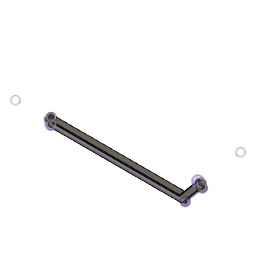
pret_collective (Autodesk Fusion 360 design; units mm, degrees)
part number: 2026-02-12-13-27-31-930
Autodesk Fusion 360 part; units mm, degrees
note: some values were not read from the file. Set by a fixed rule: which sketch regions a step uses.
sketch "Szkic1" plane through (0, 0, 0) normal (0, 1, 0) x (1, 0, 0)
  line L0 (53.834231, -5) -> (-56.165769, -5)
  line L1 (-56.165769, -5) -> (-56.165769, 0)
  line L2 (-56.165769, 0) -> (56.165769, 0)
  line L3 (0, -1.75) -> (0, -22.5)
  line L4 (1.75, 0) -> (22.5, 0)
  line L5 (53.834231, -5) -> (66.689983, -20.320889)
  line L6 (66.689983, -20.320889) -> (70.520205, -17.106951)
  line L7 (70.520205, -17.106951) -> (56.165769, 0)
  dimension "d2" = 110
  dimension "d5" = 5
  dimension "d6" = 130
  dimension "d7" = 20
  dimension "d8" = 5
  constraint perpendicular L0 L1
  constraint collinear L2 L4
  constraint perpendicular L5 L6
  constraint perpendicular L6 L7
  constraint perpendicular L1 L2
  measures "d5" distance of L5 L7
  measures "d6" angle of L0 L5
  measures "d8" distance of L0 L2
extrude "Wyciągnięcie proste1" add sketch "Szkic1" along normal mid plane 6
sketch "Szkic2" plane through (0, 0, 0) normal (0, 1, 0) x (1, 0, 0)
  circle A0 centre (69.890669, -20.246009) radius 1.7
  line L0 (70.520205, -17.106951) -> (66.689983, -20.320889)
  line L1 (68.605094, -18.71392) -> (102.400608, -58.989845)
  line L2 (56.165769, 0) -> (70.520205, -17.106951)
  line L3 (68.227373, -20.597355) -> (67.456027, -19.678101)
  line L4 (70.525506, -18.668992) -> (69.754161, -17.749738)
  line L5 (-57.365769, -4) -> (-56.165769, -4)
  circle A1 centre (-58.165769, -2.5) radius 1.7
  line L6 (-56.165769, -5) -> (-56.165769, 0)
  line L7 (-56.165769, -2.5) -> (-86.029119, -2.5)
  line L8 (-57.365769, -1) -> (-56.165769, -1)
  line L9 (-56.165769, 0) -> (56.165769, 0)
  point P0 (-56.165769, -5)
  dimension "d9" = 3.4
  dimension "d12" = 3
  dimension "d13" = 2
  dimension "d14" = 3.4
  dimension "d15" = 3
  dimension "d16" = 2
  constraint parallel L1 L2
  constraint perpendicular L0 L3
  constraint perpendicular L0 L4
  constraint symmetric L1 L3 L4
  constraint perpendicular L6 L8
  constraint perpendicular L5 L6
  constraint symmetric L5 L7 L8
  constraint vertical L6
  measures "d9" diameter of A0
  measures "d12" distance of L3 L4
  measures "d14" diameter of A1
  measures "d15" distance of L5 L8
revolve "Obrót1" add sketch "Szkic2" angle 360 about axis through (-56.165769, 0, 2.5) along (-1, 0, 0) contours L5 A1 L6 L7 | A1 L7 picked at (-56.286331, -3.151262) picked at (-58.215553, -3.147012)
revolve "Obrót2" add sketch "Szkic2" angle 360 about axis through (68.605094, 0, 18.71392) along (0.642788, 0, 0.766044) contours A0 L1 | A0 L0 L1 L3 picked at (69.144793, -20.686225) picked at (68.183694, -19.224899)
fillet "Zaokrąglenie1" radius 0.5 16 edges at (-1.165769, 3, 5) (0, 3, 0) (60.262107, -3, 12.660444) (60.262107, 3, 12.660444) (63.342987, -3, 8.553475) (63.342987, 3, 8.553475) (-1.165769, -3, 5) (0, -3, 0) (70.520205, 0, 17.106951) (68.605094, 3, 18.71392) (66.689983, 0, 20.320889) (68.605094, -3, 18.71392) (-56.165769, 0, 5) (-56.165769, -3, 2.5) (-56.165769, 0, 0) (-56.165769, 3, 2.5)
